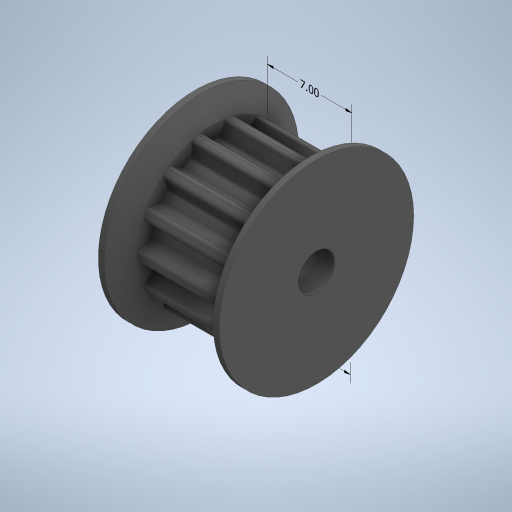
# Autodesk Inventor part: screw_gear_upper
Saved by Autodesk Inventor 2024.1 (Build 281209000, 209)
## iProperties
Category: PARTsolutions
Company: MISUMI
Created: 2025-01-17
Part Number: screw_gear_upper
Material: Generic
Catalog Web Link: www.cadenas.de
Description: HTPA__S3M060, HTPA__S3M100, HTPA__S3M150, HTPB__S3M060, HTPB__S3M100, HTPB__S3M150, HTPK__S3M060, HTPK__S3M100, HTPK__S3M150, HTPN__S3M060, HTPN__S3M100, HTPN__S3M150, HTPT__S3M060, HTPT__S3M100, HTPT__S3M150, HTPM__S3M060, HTPM__S3M100, HTPM__S3M150, HTPP__S3M060, HTPP__S3M100, HTPP__S3M150, HTPS__S3M060, HTPS__S3M100, HTPS__S3M150, KHTPA__S3M060, KHTPA__S3M100, KHTPA__S3M150, KHTPK__S3M060, KHTPK__S3M100, KHTPK__S3M150_body-High Torque Timing Pulleys S3M Type
Vendor: MISUMI
Document SubType Name: Modeling
Designer: psAdmin
Manufacturer: MISUMI
Mass: 1.12301 g
Surface Area: 12.4202 cm^2
Volume: 1.12301 cm^3
Density: 1 g/cm^3
Appearance: PSOLRGB-175-175-175
NN: 0
NT: 0
BW: 0
DD: 0
Z: 0
J: 0
Q: 0
R: 0
S: 0
T: 0
A: 0
W: 0
L: 0
PD: 0.0
OD: 0.0
D: 0
F: 0
E: 0
TT: 0
QSC: 0
QFC: 0
QTC: 0
K: 0
KSC: 0
KFC: 0
KTC: 0
ZMDD1: 0
ZMDD2: 0
ZMHH: 0
ZSC: 0
ZFC: 0
ZTC: 0
FC: 0
SRG: 0
DD2: 0
MM: 0
BTC: 0
TL: 0
BTCL: 0
BTCD: 0
BC: 0
SLH: 0
BN: 0
Title: HTPA14S3M060-A-H4
Author: Cadenas PARTsolutions
Comments: High Torque Timing Pulleys S3M Type
Autodesk Inventor part; units mm, degrees
ref_plane "YZ Plane" through (0, 0, 0) normal (1, 0, 0) x (0, 1, 0)
ref_plane "XZ Plane" through (0, 0, 0) normal (0, 1, 0) x (-1, 0, 0)
ref_plane "XY Plane" through (0, 0, 0) normal (0, 0, 1) x (1, 0, 0)
sketch "_____1" plane through (0, 0, 0) normal (0, 0, 1) x (1, 0, 0)
  line L0 (11, 0) -> (0, 0)
  line L1 (0, 0) -> (0, 5)
  line L2 (0, 5) -> (1, 5)
  line L3 (1, 5) -> (1, 6.1733)
  line L4 (1, 6.1733) -> (0.5799, 7.7412)
  line L5 (0.5799, 7.7412) -> (1.5458, 8)
  line L6 (1.5458, 8) -> (2, 6.305)
  line L7 (2, 6.305) -> (9, 6.305)
  line L8 (9, 6.305) -> (9.4542, 8)
  line L9 (9.4542, 8) -> (10.4201, 7.7412)
  line L10 (10.4201, 7.7412) -> (10, 6.1733)
  line L11 (10, 6.1733) -> (10, 5)
  line L12 (10, 5) -> (11, 5)
  line L13 (11, 5) -> (11, 0)
  line L14 (11, 0) -> (0, 0)
  constraints: 30 end point
revolve "Revolution1" add sketch "_____1" angle 360 about axis through (11, 0, 0) along (1, 0, 0)
sketch "Sketch2" plane through (11, 0, 0) normal (1, 0, 0) x (0, 0, -1)
  point P0 (0, 0)
hole "Hole1" at (11, 0, 0) direction (-1, 0, 0) diameter 4 depth 11
sketch "_____6" plane through (2, 0, 0) normal (1, 0, 0) x (0, 0, -1)
  circle A0 centre (0, 0) radius 11.305
  arc A1 (-6.3023, 0.1851) -> (-6.3023, -0.1851) centre (0, 0) ccw
  arc A2 (-6.3023, -0.1851) -> (-6.0483, -0.4556) centre (-6.0224, -0.1768) ccw
  arc A3 (-5.1954, -0.7403) -> (-6.0483, -0.4556) centre (-6.2307, -2.4222) ccw
  arc A4 (-5.126, -0.8437) -> (-5.1954, -0.7403) centre (-5.274, -0.8681) ccw
  arc A5 (-5.126, -0.8437) -> (-4.9845, -1.464) centre (0, 0) ccw
  arc A6 (-5.0021, -1.5872) -> (-4.9845, -1.464) centre (-5.1284, -1.5062) ccw
  arc A7 (-5.647, -2.2137) -> (-5.0021, -1.5872) centre (-6.6647, -0.5211) ccw
  arc A8 (-5.647, -2.2137) -> (-5.7585, -2.5677) centre (-5.5027, -2.4537) ccw
  arc A9 (-5.7585, -2.5677) -> (-5.5979, -2.9012) centre (0, 0) ccw
  arc A10 (-5.5979, -2.9012) -> (-5.2516, -3.0348) centre (-5.3493, -2.7724) ccw
  arc A11 (-4.3597, -2.9212) -> (-5.2516, -3.0348) centre (-4.5628, -4.8857) ccw
  arc A12 (-4.2523, -2.9843) -> (-4.3597, -2.9212) centre (-4.3751, -3.0704) ccw
  arc A13 (-4.2523, -2.9843) -> (-3.8557, -3.4817) centre (0, 0) ccw
  arc A14 (-3.8181, -3.6003) -> (-3.8557, -3.4817) centre (-3.967, -3.5822) ccw
  arc A15 (-4.1273, -4.4446) -> (-3.8181, -3.6003) centre (-5.7786, -3.3612) ccw
  arc A16 (-4.1273, -4.4446) -> (-4.0741, -4.8119) centre (-3.8932, -4.5982) ccw
  arc A17 (-4.0741, -4.8119) -> (-3.7847, -5.0427) centre (0, 0) ccw
  arc A18 (-3.7847, -5.0427) -> (-3.4148, -5.0128) centre (-3.6166, -4.8188) ccw
  arc A19 (-2.6605, -4.5235) -> (-3.4148, -5.0128) centre (-1.9911, -6.3816) ccw
  arc A20 (-2.5364, -4.5337) -> (-2.6605, -4.5235) centre (-2.6096, -4.6646) ccw
  arc A21 (-2.5364, -4.5337) -> (-1.9632, -4.8098) centre (0, 0) ccw
  arc A22 (-1.8779, -4.9004) -> (-1.9632, -4.8098) centre (-2.0199, -4.9486) ccw
  arc A23 (-1.7901, -5.7952) -> (-1.8779, -4.9004) centre (-3.7479, -5.5355) ccw
  arc A24 (-1.7901, -5.7952) -> (-1.5828, -6.1031) centre (-1.5125, -5.8321) ccw
  arc A25 (-1.5828, -6.1031) -> (-1.222, -6.1855) centre (0, 0) ccw
  arc A26 (-1.222, -6.1855) -> (-0.9016, -5.998) centre (-1.1677, -5.9108) ccw
  arc A27 (-0.4343, -5.2299) -> (-0.9016, -5.998) centre (0.975, -6.6135) ccw
  arc A28 (-0.3181, -5.1853) -> (-0.4343, -5.2299) centre (-0.3273, -5.335) ccw
  arc A29 (-0.3181, -5.1853) -> (0.3181, -5.1853) centre (0, 0) ccw
  arc A30 (0.4343, -5.2299) -> (0.3181, -5.1853) centre (0.3273, -5.335) ccw
  arc A31 (0.9016, -5.998) -> (0.4343, -5.2299) centre (-0.975, -6.6135) ccw
  arc A32 (0.9016, -5.998) -> (1.222, -6.1855) centre (1.1677, -5.9108) ccw
  arc A33 (1.222, -6.1855) -> (1.5828, -6.1031) centre (0, 0) ccw
  arc A34 (1.5828, -6.1031) -> (1.7901, -5.7952) centre (1.5125, -5.8321) ccw
  arc A35 (1.8779, -4.9004) -> (1.7901, -5.7952) centre (3.7479, -5.5355) ccw
  arc A36 (1.9632, -4.8098) -> (1.8779, -4.9004) centre (2.0199, -4.9486) ccw
  arc A37 (1.9632, -4.8098) -> (2.5364, -4.5337) centre (0, 0) ccw
  arc A38 (2.6605, -4.5235) -> (2.5364, -4.5337) centre (2.6096, -4.6646) ccw
  arc A39 (3.4148, -5.0128) -> (2.6605, -4.5235) centre (1.9911, -6.3816) ccw
  arc A40 (3.4148, -5.0128) -> (3.7847, -5.0427) centre (3.6166, -4.8188) ccw
  arc A41 (3.7847, -5.0427) -> (4.0741, -4.8119) centre (0, 0) ccw
  arc A42 (4.0741, -4.8119) -> (4.1273, -4.4446) centre (3.8932, -4.5982) ccw
  arc A43 (3.8181, -3.6003) -> (4.1273, -4.4446) centre (5.7786, -3.3612) ccw
  arc A44 (3.8557, -3.4817) -> (3.8181, -3.6003) centre (3.967, -3.5822) ccw
  arc A45 (3.8557, -3.4817) -> (4.2523, -2.9843) centre (0, 0) ccw
  arc A46 (4.3597, -2.9212) -> (4.2523, -2.9843) centre (4.3751, -3.0704) ccw
  arc A47 (5.2516, -3.0348) -> (4.3597, -2.9212) centre (4.5628, -4.8857) ccw
  arc A48 (5.2516, -3.0348) -> (5.5979, -2.9012) centre (5.3493, -2.7724) ccw
  arc A49 (5.5979, -2.9012) -> (5.7585, -2.5677) centre (0, 0) ccw
  arc A50 (5.7585, -2.5677) -> (5.647, -2.2137) centre (5.5027, -2.4537) ccw
  arc A51 (5.0021, -1.5872) -> (5.647, -2.2137) centre (6.6647, -0.5211) ccw
  arc A52 (4.9845, -1.464) -> (5.0021, -1.5872) centre (5.1284, -1.5062) ccw
  arc A53 (4.9845, -1.464) -> (5.126, -0.8437) centre (0, 0) ccw
  arc A54 (5.1954, -0.7403) -> (5.126, -0.8437) centre (5.274, -0.8681) ccw
  arc A55 (6.0483, -0.4556) -> (5.1954, -0.7403) centre (6.2307, -2.4222) ccw
  arc A56 (6.0483, -0.4556) -> (6.3023, -0.1851) centre (6.0224, -0.1768) ccw
  arc A57 (6.3023, -0.1851) -> (6.3023, 0.1851) centre (0, 0) ccw
  arc A58 (6.3023, 0.1851) -> (6.0483, 0.4556) centre (6.0224, 0.1768) ccw
  arc A59 (5.1954, 0.7403) -> (6.0483, 0.4556) centre (6.2307, 2.4222) ccw
  arc A60 (5.126, 0.8437) -> (5.1954, 0.7403) centre (5.274, 0.8681) ccw
  arc A61 (5.126, 0.8437) -> (4.9845, 1.464) centre (0, 0) ccw
  arc A62 (5.0021, 1.5872) -> (4.9845, 1.464) centre (5.1284, 1.5062) ccw
  arc A63 (5.647, 2.2137) -> (5.0021, 1.5872) centre (6.6647, 0.5211) ccw
  arc A64 (5.647, 2.2137) -> (5.7585, 2.5677) centre (5.5027, 2.4537) ccw
  arc A65 (5.7585, 2.5677) -> (5.5979, 2.9012) centre (0, 0) ccw
  arc A66 (5.5979, 2.9012) -> (5.2516, 3.0348) centre (5.3493, 2.7724) ccw
  arc A67 (4.3597, 2.9212) -> (5.2516, 3.0348) centre (4.5628, 4.8857) ccw
  arc A68 (4.2523, 2.9843) -> (4.3597, 2.9212) centre (4.3751, 3.0704) ccw
  arc A69 (4.2523, 2.9843) -> (3.8557, 3.4817) centre (0, 0) ccw
  arc A70 (3.8181, 3.6003) -> (3.8557, 3.4817) centre (3.967, 3.5822) ccw
  arc A71 (4.1273, 4.4446) -> (3.8181, 3.6003) centre (5.7786, 3.3612) ccw
  arc A72 (4.1273, 4.4446) -> (4.0741, 4.8119) centre (3.8932, 4.5982) ccw
  arc A73 (4.0741, 4.8119) -> (3.7847, 5.0427) centre (0, 0) ccw
  arc A74 (3.7847, 5.0427) -> (3.4148, 5.0128) centre (3.6166, 4.8188) ccw
  arc A75 (2.6605, 4.5235) -> (3.4148, 5.0128) centre (1.9911, 6.3816) ccw
  arc A76 (2.5364, 4.5337) -> (2.6605, 4.5235) centre (2.6096, 4.6646) ccw
  arc A77 (2.5364, 4.5337) -> (1.9632, 4.8098) centre (0, 0) ccw
  arc A78 (1.8779, 4.9004) -> (1.9632, 4.8098) centre (2.0199, 4.9486) ccw
  arc A79 (1.7901, 5.7952) -> (1.8779, 4.9004) centre (3.7479, 5.5355) ccw
  arc A80 (1.7901, 5.7952) -> (1.5828, 6.1031) centre (1.5125, 5.8321) ccw
  arc A81 (1.5828, 6.1031) -> (1.222, 6.1855) centre (0, 0) ccw
  arc A82 (1.222, 6.1855) -> (0.9016, 5.998) centre (1.1677, 5.9108) ccw
  arc A83 (0.4343, 5.2299) -> (0.9016, 5.998) centre (-0.975, 6.6135) ccw
  arc A84 (0.3181, 5.1853) -> (0.4343, 5.2299) centre (0.3273, 5.335) ccw
  arc A85 (0.3181, 5.1853) -> (-0.3181, 5.1853) centre (0, 0) ccw
  arc A86 (-0.4343, 5.2299) -> (-0.3181, 5.1853) centre (-0.3273, 5.335) ccw
  arc A87 (-0.9016, 5.998) -> (-0.4343, 5.2299) centre (0.975, 6.6135) ccw
  arc A88 (-0.9016, 5.998) -> (-1.222, 6.1855) centre (-1.1677, 5.9108) ccw
  arc A89 (-1.222, 6.1855) -> (-1.5828, 6.1031) centre (0, 0) ccw
  arc A90 (-1.5828, 6.1031) -> (-1.7901, 5.7952) centre (-1.5125, 5.8321) ccw
  arc A91 (-1.8779, 4.9004) -> (-1.7901, 5.7952) centre (-3.7479, 5.5355) ccw
  arc A92 (-1.9632, 4.8098) -> (-1.8779, 4.9004) centre (-2.0199, 4.9486) ccw
  arc A93 (-1.9632, 4.8098) -> (-2.5364, 4.5337) centre (0, 0) ccw
  arc A94 (-2.6605, 4.5235) -> (-2.5364, 4.5337) centre (-2.6096, 4.6646) ccw
  arc A95 (-3.4148, 5.0128) -> (-2.6605, 4.5235) centre (-1.9911, 6.3816) ccw
  arc A96 (-3.4148, 5.0128) -> (-3.7847, 5.0427) centre (-3.6166, 4.8188) ccw
  arc A97 (-3.7847, 5.0427) -> (-4.0741, 4.8119) centre (0, 0) ccw
  arc A98 (-4.0741, 4.8119) -> (-4.1273, 4.4446) centre (-3.8932, 4.5982) ccw
  arc A99 (-3.8181, 3.6003) -> (-4.1273, 4.4446) centre (-5.7786, 3.3612) ccw
  arc A100 (-3.8557, 3.4817) -> (-3.8181, 3.6003) centre (-3.967, 3.5822) ccw
  arc A101 (-3.8557, 3.4817) -> (-4.2523, 2.9843) centre (0, 0) ccw
  arc A102 (-4.3597, 2.9212) -> (-4.2523, 2.9843) centre (-4.3751, 3.0704) ccw
  arc A103 (-5.2516, 3.0348) -> (-4.3597, 2.9212) centre (-4.5628, 4.8857) ccw
  arc A104 (-5.2516, 3.0348) -> (-5.5979, 2.9012) centre (-5.3493, 2.7724) ccw
  arc A105 (-5.5979, 2.9012) -> (-5.7585, 2.5677) centre (0, 0) ccw
  arc A106 (-5.7585, 2.5677) -> (-5.647, 2.2137) centre (-5.5027, 2.4537) ccw
  arc A107 (-5.0021, 1.5872) -> (-5.647, 2.2137) centre (-6.6647, 0.5211) ccw
  arc A108 (-4.9845, 1.464) -> (-5.0021, 1.5872) centre (-5.1284, 1.5062) ccw
  arc A109 (-4.9845, 1.464) -> (-5.126, 0.8437) centre (0, 0) ccw
  arc A110 (-5.1954, 0.7403) -> (-5.126, 0.8437) centre (-5.274, 0.8681) ccw
  arc A111 (-6.0483, 0.4556) -> (-5.1954, 0.7403) centre (-6.2307, 2.4222) ccw
  arc A112 (-6.0483, 0.4556) -> (-6.3023, 0.1851) centre (-6.0224, 0.1768) ccw
  constraints: 224 point on circle, 113 centre point
extrude "Extrusion1" cut sketch "_____6" along normal blind 7
ref_plane "to_belt_XY" through (5.5, 0, 0) normal (-1, 0, 0) x (0, 0, -1)
ref_plane "to_belt_YZ" through (5.5, 0, 0) normal (0, 0, -1) x (0, -1, 0)
ref_plane "to_belt_ZX" through (5.5, 0, 0) normal (0, -1, 0) x (-1, 0, 0)
sketch "スケッチ4" plane through (11, 0, 0) normal (1, 0, 0) x (0, 0, -1)
  circle A0 centre (0, 0) radius 8 projected
extrude "押し出し2" cut sketch "スケッチ4" against normal up to surface (2 mm away)
ref_plane "作業平面4" through (5.5, 0, 0) normal (1, 0, 0) x (0, 0, -1)
sketch "スケッチ5" plane through (9, 0, 0) normal (1, 0, 0) x (0, 0, -1)
  circle A0 centre (0, 0) radius 6.305
  arc A1 (5.7585, -2.5677) -> (6.3023, -0.1851) centre (0, 0) ccw projected
  circle A2 centre (0, 0) radius 2 projected
  constraints: 1 centre point, 1 coincident, 1 concentric
extrude "押し出し3" add sketch "スケッチ5" along normal blind 1 draft 60 contours A0 | A2
sketch "スケッチ6" plane through (10, 0, 0) normal (1, 0, 0) x (0, 0, -1)
  circle A0 centre (0, 0) radius 8.0371 projected
extrude "押し出し4" add sketch "スケッチ6" along normal blind 0.5
sketch "スケッチ8" plane through (9, 0, 0) normal (-1, 0, 0) x (0, 0, 1)
  circle A0 centre (0, 0) radius 2 projected
extrude "押し出し6" add sketch "スケッチ8" along normal blind 3.5
sketch "スケッチ9" plane through (10.5, 0, 0) normal (1, 0, 0) x (0, 0, -1)
  circle A0 centre (0, 0) radius 1.5
  dimension "d22" = 3
  constraints: 1 centre point, 1 coincident
  measures "d22" diameter of A0
extrude "押し出し7" cut sketch "スケッチ9" against normal through all
mirror "ミラー1" about plane through (5.5, 0, 0) normal (1, 0, 0) of "押し出し2", "押し出し3", "押し出し4", "押し出し6", "押し出し7"
sketch "スケッチ10" plane through (0.5, 0, 0) normal (-1, 0, 0) x (0, 0, 1)
  circle A0 centre (0, 0) radius 5
  dimension "d28" = 10
  constraints: 1 centre point, 1 coincident
  measures "d28" diameter of A0
extrude "押し出し8" cut sketch "スケッチ10" against normal blind 3.2
sketch "スケッチ12" plane through (0, 0, 0) normal (0, 1, 0) x (-1, 0, 0)
  line L0 (-3.7, -1.5) -> (-3.7, 1.5) projected
  line L1 (-10.5, -1.5) -> (-10.5, 1.5) projected
  line L2 (-10.5, 0) -> (-3.7, 0)
  circle A0 centre (-7.1, 0) radius 0.85
  point P0 (0, 0)
  dimension "d34" = 1.7
  constraints: 3 midpoint, 2 end point, 1 centre point
  measures "d34" diameter of A0
extrude "押し出し10" cut sketch "スケッチ12" against normal through all
body "Solid1"
